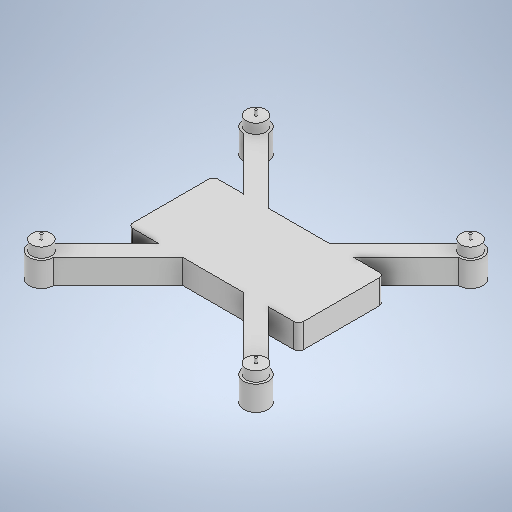
# Autodesk Inventor part: DroneBase
Saved by Autodesk Inventor 2025.1 (Build 291241000, 241)
## iProperties
Created: 2024-10-02
Part Number: DroneBase
Material: Generic
Document SubType Name: Modeling
Designer: fears
Density: 1 g/cm^3
Appearance: Default
Author: fears
Autodesk Inventor part; units mm, degrees
ref_plane "YZ Plane" through (0, 0, 0) normal (1, 0, 0) x (0, 1, 0)
ref_plane "XZ Plane" through (0, 0, 0) normal (0, 1, 0) x (-1, 0, 0)
ref_plane "XY Plane" through (0, 0, 0) normal (0, 0, 1) x (1, 0, 0)
sketch "Sketch1" plane through (0, 0, 0) normal (0, 1, 0) x (-1, 0, 0)
  line L0 (49, 49) -> (-49, 49)
  line L1 (-49, 49) -> (-49, -49)
  line L2 (-49, -49) -> (49, -49)
  line L3 (49, -49) -> (49, 49)
  line L4 (49, 49) -> (-49, -49)
  line L5 (49, -49) -> (-49, 49)
  circle A0 centre (44, 44) radius 5
  line L6 (0, 0) -> (0, 5)
  line L7 (0, 0) -> (5, 0)
  line L8 (5, 0) -> (44, 39)
  line L9 (39, 44) -> (0, 5)
  circle A1 centre (-44, 44) radius 5
  line L10 (-44, 39) -> (-5, 0)
  line L11 (0, 5) -> (-39, 44)
  circle A2 centre (-44, -44) radius 5
  line L12 (-39, -44) -> (0, -5)
  line L13 (-5, 0) -> (-44, -39)
  circle A3 centre (44, -44) radius 5
  line L14 (44, -39) -> (5, 0)
  line L15 (0, -5) -> (39, -44)
  line L16 (-33, 17.5) -> (33, 17.5)
  line L17 (35, 15.5) -> (35, -15.5)
  line L18 (33, -17.5) -> (-33, -17.5)
  line L19 (-35, -15.5) -> (-35, 15.5)
  line L20 (-35, 17.5) -> (35, -17.5) construction
  line L21 (35, 17.5) -> (-35, -17.5) construction
  arc A4 (35, 15.5) -> (33, 17.5) centre (33, 15.5) ccw
  arc A5 (33, -17.5) -> (35, -15.5) centre (33, -15.5) ccw
  arc A6 (-35, -15.5) -> (-33, -17.5) centre (-33, -15.5) ccw
  arc A7 (-33, 17.5) -> (-35, 15.5) centre (-33, 15.5) ccw
  point P0 (12.5, 17.5)
  point P1 (-12.5, 17.5)
  point P2 (-22.5, 17.5)
  point P3 (-22.5, -17.5)
  point P4 (-12.5, -17.5)
  point P5 (12.5, -17.5)
  point P6 (22.5, -17.5)
  point P7 (22.5, 17.5)
  dimension "d0" = 98
  dimension "d1" = 98
  dimension "d2" = 10
  dimension "d3" = 49
  dimension "d4" = 49
  dimension "d7" = 360
  dimension "d10" = 70
  dimension "d11" = 35
  dimension "d12" = 2
  dimension "d13" = 2
  dimension "d14" = 2
  dimension "d15" = 2
  constraints: 44 end point, 16 point on circle, 9 point on line, 9 tangent, 8 centre point, 4 parallel, 3 perpendicular, 2 horizontal, 2 midpoint, 1 vertical, 33 other
  measures "d0" distance of L2.end L0.start
  measures "d1" distance of L0.start L0.end
  measures "d2" diameter of A0
  measures "d3" horizontal distance of L6.start L0.start
  measures "d4" horizontal distance of L6.start L0.start
  measures "d10" distance of L20.end L21.end
  measures "d11" distance of L21.start L20.end
  measures "d12" radius of A4
  measures "d13" radius of A5
  measures "d14" radius of A6
  measures "d15" radius of A7
extrude "Extrusion1" add sketch "Sketch1" along normal blind 10 contours A0 L4 | A0 L4 | A1 L5 | A0 L4 L16 L9 | A3 L5 | L8 L16 L4 A0 | L11 L16 L5 A1 | L5 A1 | L16 L4 L6 L9 | L9 L11 L16 | A3 L5 L18 L14 | A3 L5 | L16 A4 L17 A5 L18 L14 L8 | L8 L7 L4 L16 | L5 L16 L10 A1 | L11 L6 L5 L16 | A3 L15 L18 L5 | L18 L5 L7 L14 | L5 L18 L15 L12 L4 | L4 L18 L13 L10 L16 L5 | A2 L4 | A2 L4 | L18 L12 A2 L4 | L4 A2 L13 L18 | L10 L13 L18 A6 L19 A7 L16 | L18 L12 L15
sketch "Sketch2" plane through (0, 10, 0) normal (0, 1, 0) x (1, 0, 0)
  arc A0 (-44, -39) -> (-39, -44) centre (-44, -44) ccw projected
  circle A1 centre (-44, -44) radius 4
  arc A2 (-39, 44) -> (-44, 39) centre (-44, 44) ccw projected
  circle A3 centre (-44, 44) radius 4
  arc A4 (44, 39) -> (39, 44) centre (44, 44) ccw projected
  circle A5 centre (44, 44) radius 4
  arc A6 (39, -44) -> (44, -39) centre (44, -44) ccw projected
  circle A7 centre (44, -44) radius 4
  point P0 (0, 0)
  dimension "d18" = 8
  dimension "d19" = 8
  dimension "d20" = 8
  dimension "d21" = 8
  constraints: 4 centre point, 4 coincident
  measures "d18" diameter of A1
  measures "d19" diameter of A3
  measures "d20" diameter of A5
  measures "d21" diameter of A7
extrude "Extrusion2" add sketch "Sketch2" along normal blind 4
sketch "Sketch3" plane through (-44, 14, 44) normal (0, 1, 0) x (1, 0, 0)
  circle A0 centre (0, 0) radius 0.5
  point P0 (44, 44)
  dimension "d24" = 1
  constraints: 1 centre point
  measures "d24" diameter of A0
sketch "Sketch4" plane through (-44, 14, -44) normal (0, 1, 0) x (1, 0, 0)
  circle A0 centre (0, 0) radius 4 projected
  circle A1 centre (0, 0) radius 0.5
  point P0 (44, -44)
  dimension "d25" = 1
  constraints: 1 centre point, 1 coincident
  measures "d25" diameter of A1
sketch "Sketch5" plane through (44, 14, -44) normal (0, 1, 0) x (1, 0, 0)
  circle A0 centre (0, 0) radius 4 projected
  circle A1 centre (0, 0) radius 0.5
  point P0 (-44, -44)
  dimension "d26" = 1
  constraints: 1 centre point, 1 coincident
  measures "d26" diameter of A1
sketch "Sketch6" plane through (44, 14, 44) normal (0, 1, 0) x (1, 0, 0)
  circle A0 centre (0, 0) radius 4 projected
  circle A1 centre (0, 0) radius 0.5
  point P0 (-44, 44)
  dimension "d27" = 1
  constraints: 1 centre point, 1 coincident
  measures "d27" diameter of A1
extrude "Extrusion3" add sketch "Sketch6" along normal blind 2 contours A1
extrude "Extrusion4" add sketch "Sketch3" along normal blind 2
extrude "Extrusion5" add sketch "Sketch4" along normal blind 2 contours A1
extrude "Extrusion6" add sketch "Sketch5" along normal blind 2 contours A1
body "Solid1"
